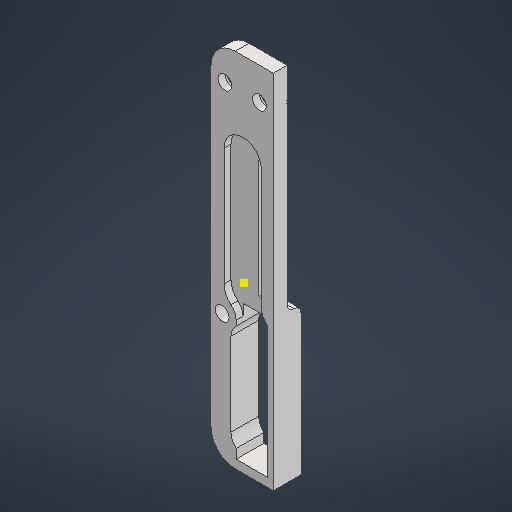
# Autodesk Inventor part: 指纹安装板
Saved by Autodesk Inventor 2025 (Build 290162000, 162)
## iProperties
Created: 2025-11-30
Part Number: 指纹安装板
Material: 常规
Document SubType Name: Modeling
Designer: XH
Density: 1 g/cm^3
Appearance: 默认
Author: XH
Autodesk Inventor part; units mm, degrees
ref_plane "YZ Plane" through (0, 0, 0) normal (1, 0, 0) x (0, 1, 0)
ref_plane "XZ Plane" through (0, 0, 0) normal (0, 1, 0) x (-1, 0, 0)
ref_plane "XY Plane" through (0, 0, 0) normal (0, 0, 1) x (1, 0, 0)
sketch "草图1" plane through (0, 0, 0) normal (0, 0, 1) x (1, 0, 0)
  point P0 (0, 0)
sketch "草图2" plane through (0, 0, 0) normal (0, 0, 1) x (1, 0, 0)
  arc A0 (-0.8636, -19.593) -> (1.5364, -19.593) centre (0.3364, -19.593) ccw
  line L0 (-0.8636, -19.593) -> (-0.8636, -7.593)
  arc A1 (1.5364, -7.593) -> (-0.8636, -7.593) centre (0.3364, -7.593) ccw
  line L1 (1.5364, -7.593) -> (1.5364, -19.593)
  arc A2 (-1.8636, -1.5566) -> (1.5364, -1.5566) centre (-0.1636, -1.5566) ccw
  line L2 (-1.8636, 15.4434) -> (-1.8636, -1.5566)
  arc A3 (1.5364, 15.4434) -> (-1.8636, 15.4434) centre (-0.1636, 15.4434) ccw
  line L3 (1.5364, 8.4451) -> (1.5364, 15.4434)
  arc A4 (1.3364, 8.2451) -> (1.5364, 8.4451) centre (1.3364, 8.4451) ccw
  line L4 (1.3364, 8.2451) -> (1.2785, 8.2451)
  arc A5 (1.0785, 8.4451) -> (1.2785, 8.2451) centre (1.2785, 8.4451) ccw
  line L5 (1.0785, 8.4451) -> (1.0785, 15.3461)
  arc A6 (1.0785, 15.3461) -> (-1.3205, 15.3461) centre (-0.121, 15.3461) ccw
  line L6 (-1.3205, 15.3461) -> (-1.3205, -1.4976)
  arc A7 (-1.3205, -1.4976) -> (1.0785, -1.4976) centre (-0.121, -1.4976) ccw
  line L7 (1.0785, -1.4976) -> (1.0785, 5.4033)
  arc A8 (1.2785, 5.6033) -> (1.0785, 5.4033) centre (1.2785, 5.4033) ccw
  line L8 (1.2785, 5.6033) -> (1.3364, 5.6033)
  arc A9 (1.5364, 5.4033) -> (1.3364, 5.6033) centre (1.3364, 5.4033) ccw
  line L9 (1.5364, -1.5566) -> (1.5364, 5.4033)
  arc A10 (-4.7477, -20.3592) -> (-3.3007, -23.1939) centre (-1.2477, -20.3592) ccw
  spline S0 degree 3 poles (-1.2477, -23.8592) (-1.6067, -23.8592) (-1.9735, -23.8009) (-2.735, -23.5583) (-3.0595, -23.3686) (-3.3007, -23.1939) knots 0 0 0 0 0.450925 0.450925 1 1 1 1
  line L10 (5.2523, -23.8592) -> (-1.2477, -23.8592)
  line L11 (5.2523, 28.3531) -> (5.2523, -23.8592)
  line L12 (-1.2477, 28.3531) -> (5.2523, 28.3531)
  arc A11 (-1.2477, 28.3531) -> (-4.7477, 24.8531) centre (-1.2477, 24.8531) ccw
  line L13 (-4.7477, -20.3592) -> (-4.7477, 24.8531)
  line L14 (4.2523, -23.8592) -> (4.2523, 28.3531)
  line L15 (5.2523, 28.3531) -> (4.2523, 28.3531)
  line L16 (5.2523, -23.8592) -> (5.2523, 28.3531)
  line L17 (4.2523, -23.8592) -> (5.2523, -23.8592)
  point P0 (0, 0)
extrude "拉伸1" add sketch "草图2" along normal blind 4 contours L0 A1 L1 A0 | L2 A3 L3 A4 L4 A5 L5 A6 L6 A7 L7 A8 L8 A9 L9 A2 | L13 A11 L12 L14 L10 S0 A10
sketch "草图3" plane through (0, 0, 4) normal (0, 0, 1) x (1, 0, 0)
  point P0 (0, 0)
sketch "草图4" plane through (0, 0, 0) normal (0, 0, -1) x (-1, 0, 0)
  line L0 (-3.3928, -22.593) -> (-3.3928, -3.4829)
  line L1 (-3.3928, -3.4829) -> (-4.2523, -3.4829)
  line L2 (-4.2523, -3.4829) -> (-4.2523, -23.8592)
  line L3 (-4.2523, -23.8592) -> (1.2477, -23.8592)
  spline S0 degree 3 poles (1.2477, -23.8592) (1.6878, -23.8592) (2.1571, -23.7712) (2.6422, -23.5699) (2.6953, -23.5463) (2.7477, -23.5215) knots 0 0 0 0 0.889543 0.889543 1 1 1 1
  line L4 (2.7477, -23.5215) -> (2.7477, -3.4829)
  line L5 (2.7477, -3.4829) -> (1.1072, -3.4829)
  line L6 (1.1072, -3.4829) -> (1.1072, -5.9329)
  arc A0 (1.8636, -7.593) -> (1.1072, -5.9329) centre (-0.3364, -7.593) ccw
  line L7 (1.8636, -7.593) -> (1.8636, -19.593)
  arc A1 (1.1072, -21.2531) -> (1.8636, -19.593) centre (-0.3364, -19.593) ccw
  line L8 (1.1072, -21.2531) -> (1.1072, -22.593)
  line L9 (1.1072, -22.593) -> (-3.3928, -22.593)
  line L10 (1.1072, -3.593) -> (-3.3928, -3.593)
  point P0 (0, 0)
extrude "拉伸2" cut sketch "草图4" against normal blind 4 contours L0 L10 L6 A0 L7 A1 L8 L9
sketch "草图5" plane through (0, 0, 0) normal (0, 0, -1) x (-1, 0, 0)
  line L0 (-2.3928, -3.593) -> (-2.3928, -22.593) projected
  line L1 (-2.3928, -3.593) -> (-3.3928, -3.593) projected
  line L2 (-3.3928, -22.593) -> (-3.3928, -3.593) projected
  line L3 (-2.3928, -22.593) -> (-3.3928, -22.593) projected
  point P0 (0, 0)
extrude "拉伸3" add sketch "草图5" against normal blind 2
sketch "草图6" plane through (4.2523, -23.8592, 0) normal (1, 0, 0) x (0, 0, -1)
  line L0 (0.0883, 54.0026) -> (-2, 54.0026)
  line L1 (-2, 54.0026) -> (-2, 21.2662)
  line L2 (-2, 21.2662) -> (0.0883, 21.2662)
  line L3 (0.0883, 21.2662) -> (0.0883, 54.0026)
  line L4 (1, 20.2662) -> (-3, 20.2662) projected
  line L5 (-4, 0) -> (-4, 52.2123) projected
  point P0 (0, 23.8592)
  point P1 (-1, 20.2662)
  dimension "d6" = 1
  dimension "d7" = 2
  constraints: 8 end point, 2 parallel, 1 horizontal, 1 midpoint, 1 perpendicular
  measures "d6" distance from line of point (-1, 20.266) L2
  measures "d7" distance between parallel lines of L5 L1
extrude "拉伸4" cut sketch "草图6" against normal blind 33
fillet "圆角1" radius 1 2 edges at (-0.2477, -2.593, 2) (-0.2477, -2.593, 0)
sketch "草图7" plane through (0, 0, 4) normal (0, 0, 1) x (1, 0, 0)
  arc A0 (-1.8636, -1.5566) -> (1.5364, -1.5566) centre (-0.1636, -1.5566) ccw projected
  line L0 (-1.8636, 15.4434) -> (-1.8636, -1.5566) projected
  line L1 (1.5364, -1.5566) -> (1.5364, 5.4033) projected
  line L2 (1.379, -1.5758) -> (1.379, 15.4242) projected
  arc A1 (1.5364, 15.4434) -> (-1.8636, 15.4434) centre (-0.1636, 15.4434) ccw projected
  line L3 (1.5364, -1.5566) -> (1.5364, 15.4434) projected
  line L4 (-2.8636, 15.4434) -> (-2.8636, -1.5566)
  arc A2 (-2.8636, -1.5566) -> (2.5364, -1.5566) centre (-0.1636, -1.5566) ccw
  line L5 (2.5364, -1.5566) -> (2.5364, 15.4434)
  arc A3 (2.5364, 15.4434) -> (-2.8636, 15.4434) centre (-0.1636, 15.4434) ccw
  point P0 (0, 0)
  dimension "d11" = 1
  constraints: 4 end point, 4 point on circle, 2 centre point, 3 other
  measures "d11" radial gap between concentric circles of A1 A3
extrude "拉伸5" cut sketch "草图7" against normal blind 1 contours L0 A1 L3 L1 A0 | A3 L5 A2 L4
fillet "圆角2" radius 2 2 edges at (-1.1072, -4.0864, 3.5) (1.6093, -3.593, 3.5)
sketch "草图8" plane through (0, 0, 3) normal (0, 0, 1) x (1, 0, 0)
  arc A0 (2.5364, 15.4434) -> (-2.8636, 15.4434) centre (-0.1636, 15.4434) ccw projected
  line L0 (2.5364, 15.4434) -> (1.1862, 15.4434)
  line L1 (1.1862, 15.4434) -> (1.1862, -1.593)
  line L2 (1.1862, -1.593) -> (2.5364, -1.593)
  line L3 (2.5364, -1.593) -> (2.5364, 15.4434)
  line L4 (-4.7477, -1.593) -> (4.2523, -1.593) projected
  point P0 (0, 0)
  constraints: 8 end point, 2 parallel, 1 collinear, 1 horizontal, 1 perpendicular
extrude "拉伸6" cut sketch "草图8" against normal blind 1
sketch "草图9" plane through (0, 0, 4) normal (0, 0, 1) x (1, 0, 0)
  point P0 (0, 0)
sketch "草图10" plane through (0, 0, 4) normal (0, 0, 1) x (1, 0, 0)
  circle A0 centre (-2.7477, 23.7142) radius 1
  circle A1 centre (2.2523, 23.7142) radius 1
  line L0 (4.2523, -23.8592) -> (4.2523, 28.3531) projected
  line L1 (-4.7477, 24.8531) -> (-4.7477, -20.3592) projected
  circle A2 centre (-3.1277, -5.3622) radius 1
  point P0 (0, 0)
  dimension "d17" = 2
  dimension "d18" = 2
  dimension "d19" = 2
  dimension "d20" = 2
  dimension "d21" = 2
  constraints: 3 centre point, 1 horizontal alignment
  measures "d17" diameter of A0
  measures "d18" diameter of A1
  measures "d19" distance from line of L0 A1.centre
  measures "d20" distance from line of A0.centre L1
  measures "d21" diameter of A2
extrude "拉伸7" cut sketch "草图10" against normal blind 9.5
chamfer "倒角1" distance 1 angle 45 3 edges at (-3.7477, 23.7142, 2) (1.2523, 23.7142, 2) (-4.1277, -5.3622, 0)
